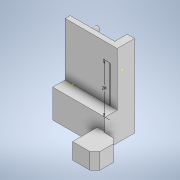
# Autodesk Inventor part: base_fin_carrera
Saved by Autodesk Inventor 2021 (Build 250183000, 183)
## iProperties
Created: 2021-05-13
Part Number: base_fin_carrera
Material: Genérico
Document SubType Name: Modeling
Designer: orgyn
Density: 1 g/cm^3
Appearance: Valor por defecto
Author: orgyn
Autodesk Inventor part; units mm, degrees
ref_plane "YZ Plane" through (0, 0, 0) normal (1, 0, 0) x (0, 1, 0)
ref_plane "XZ Plane" through (0, 0, 0) normal (0, 1, 0) x (-1, 0, 0)
sketch "Boceto1" plane through (0, 0, 0) normal (0, 1, 0) x (-1, 0, 0)
  line L0 (0, 0) -> (-4, 0)
  line L1 (-4, 0) -> (-4, -9.5)
  line L2 (-4, -9.5) -> (0, -9.5)
  line L3 (0, -9.5) -> (0, 0)
  dimension "d0" = 4
  dimension "d1" = 9.5
  constraints: 8 end point, 2 parallel, 1 horizontal, 1 perpendicular
  measures "d0" distance of L2.end L1.end
  measures "d1" distance of L1.end L0.end
extrude "Extrusión1" add sketch "Boceto1" along normal blind 4
sketch "Boceto2" plane through (0, 0, -9.5) normal (-1, 0, 0) x (0, 0, 1)
  line L0 (9.5, 4) -> (0, 4) projected
  line L1 (9.5, 4) -> (-4.5, 4)
  line L2 (-4.5, 4) -> (-7.5, 4)
  line L3 (-5, 0) -> (-5, -16)
  line L4 (0, 0) -> (0, 4) projected
  line L5 (9.5, 0) -> (0, 0) projected
  line L6 (0, 0) -> (9.5, 0)
  line L7 (9.5, 0) -> (9.5, 4)
  line L8 (-5, -16) -> (-12.5, -16)
  line L9 (-12.5, -16) -> (-12.5, 4)
  line L10 (-12.5, 4) -> (-7.5, 4)
  line L11 (-5, 0) -> (9.5, 0)
  line L12 (-5, 4) -> (9.5, 4)
  line L13 (9.5, 0) -> (9.5, 4) projected
  line L14 (9.5, 0) -> (9.5, 4)
  dimension "d4" = 14
  dimension "d5" = 3
  dimension "d6" = 20
  dimension "d25" = 7.5
  constraints: 22 end point, 4 collinear, 3 horizontal, 3 perpendicular
  measures "d4" distance of L0.start L1.end
  measures "d5" distance of L2.end L1.end
  measures "d6" distance of L12.start L3.end
  measures "d25" distance of L8.start L8.end
extrude "Extrusión2" add sketch "Boceto2" along normal blind 2 contours L7 L5 L4 L0
sketch "Boceto3" plane through (-2, 0, -9.5) normal (-1, 0, 0) x (0, 0, 1)
  line L0 (9.5, 4) -> (0, 4) projected
  line L1 (-7.5, 4) -> (-2.5, 4)
  line L2 (-2.5, 4) -> (-2.5, 1.5)
  line L3 (-2.5, 1.5) -> (-7.5, 1.5)
  line L4 (-7.5, 4) -> (-7.5, -16) projected
  line L5 (-7.5, 1.5) -> (-7.5, -4.5)
  line L6 (-7.5, -4.5) -> (-7.5, -10.5)
  line L7 (-7.5, -10.5) -> (-7.5, -13)
  line L8 (-7.5, -13) -> (-2.5, -13)
  line L9 (-2.5, -13) -> (-2.5, -10.5)
  line L10 (-2.5, -10.5) -> (-7.5, -10.5)
  line L11 (-7.5, -4.5) -> (-7.5, -5.75)
  line L12 (-7.5, -5.75) -> (-2.5, -5.75)
  line L13 (-2.5, -5.75) -> (-2.5, -3.25)
  line L14 (-2.5, -3.25) -> (-7.5, -3.25)
  point P0 (9.5, 0)
  dimension "d9" = 5
  dimension "d10" = 2.5
  dimension "d11" = 6
  dimension "d12" = 6
  dimension "d13" = 2.5
  dimension "d14" = 5
  dimension "d15" = 2.5
  dimension "d16" = 1.25
  dimension "d17" = 5
  dimension "d18" = 2.5
  constraints: 26 end point, 9 point on line, 4 perpendicular, 1 parallel
  measures "d9" distance of L1.start L1.end
  measures "d10" distance of L1.end L2.end
  measures "d11" distance of L3.end L5.end
  measures "d12" distance of L5.end L6.end
  measures "d13" distance of L6.end L7.end
  measures "d14" distance of L7.end L8.end
  measures "d15" distance of L8.end L9.end
  measures "d16" distance of L5.end L11.end
  measures "d17" distance of L11.end L12.end
  measures "d18" distance of L12.end L13.end
extrude "Extrusión3" cut sketch "Boceto3" against normal blind 1
chamfer "Chaflán1" distance 2 angle 45 2 edges at (4, 2, -9.5) (4, 2, 0)
sketch "Boceto4" plane through (-2, 0, -9.5) normal (-1, 0, 0) x (0, 0, 1)
  line L0 (0, 0) -> (9.5, 0) projected
  line L1 (9.5, 0) -> (0, 0)
  line L2 (0, 0) -> (-5, 0)
  line L3 (-5, 0) -> (-5, -20)
  line L4 (-5, -20) -> (-12.5, -20)
  line L5 (-12.5, -20) -> (-12.5, 4)
  line L6 (9.5, 4) -> (0, 4) projected
  line L7 (-12.5, 4) -> (9.5, 4)
  line L8 (9.5, 0) -> (9.5, 4) projected
  line L9 (9.5, 4) -> (9.5, 0)
  line L10 (-12.5, 4) -> (-7.5, 4)
  line L11 (-7.5, 4) -> (-7.5, 1.5)
  line L12 (-7.5, 1.5) -> (-12.5, 1.5)
  line L13 (-12.5, 1.2493) -> (-12.5, -4.7507)
  line L14 (-12.5, -4.7507) -> (-12.5, -10.7507)
  line L15 (-12.5, -10.7507) -> (-7.5, -10.7507)
  line L16 (-7.5, -10.7507) -> (-7.5, -13.2507)
  line L17 (-7.5, -13.2507) -> (-12.5, -13.2507)
  line L18 (-12.5, -4.7507) -> (-12.5, -6.0007)
  line L19 (-12.5, -6.0007) -> (-7.5, -6.0007)
  line L20 (-7.5, -6.0007) -> (-7.5, -3.5007)
  line L21 (-7.5, -3.5007) -> (-12.5, -3.5007)
  dimension "d26" = 5
  dimension "d27" = 20
  dimension "d28" = 7.5
  dimension "d29" = 5
  dimension "d30" = 2.5
  dimension "d31" = 6
  dimension "d32" = 6
  dimension "d33" = 5
  dimension "d34" = 2.5
  dimension "d35" = 1.25
  dimension "d36" = 2.5
  constraints: 38 end point, 13 point on line, 8 perpendicular, 3 collinear
  measures "d26" distance of L0.start L2.end
  measures "d27" distance of L2.end L3.end
  measures "d28" distance of L3.end L4.end
  measures "d29" distance of L5.end L10.end
  measures "d30" distance of L10.end L11.end
  measures "d31" distance of L13.start L13.end
  measures "d32" distance of L13.end L14.end
  measures "d33" distance of L14.end L15.end
  measures "d34" distance of L15.end L16.end
  measures "d35" distance of L13.end L18.end
  measures "d36" distance of L19.end L20.end
extrude "Extrusión4" add sketch "Boceto4" along normal blind 3 contours L2 L3 L4 L5 L17 L16 L15 L19 L20 L21 L12 L11 L7 L6 L8 L0
sketch "Boceto5" plane through (0, 4, 0) normal (0, 1, 0) x (1, 0, 0)
  line L0 (-2, 17) -> (-5, 17) projected
  line L1 (-5, 17) -> (-2, 17)
  line L2 (-2, 14.5) -> (-2, 9.5) projected
  line L3 (-2, 17) -> (-2, 9.5)
  line L4 (2, 9.5) -> (-2, 9.5) projected
  line L5 (-2, 9.5) -> (2, 9.5)
  line L6 (4, 7.5) -> (2, 9.5) projected
  line L7 (2, 9.5) -> (4, 7.5)
  line L8 (4, 2) -> (4, 7.5) projected
  line L9 (4, 7.5) -> (4, 2)
  line L10 (2, 0) -> (4, 2) projected
  line L11 (4, 2) -> (2, 0)
  line L12 (2, 0) -> (-5, 0) projected
  line L13 (2, 0) -> (-5, 0)
  line L14 (-5, 0) -> (-5, 17) projected
  line L15 (-5, 0) -> (-5, 17)
  point P0 (0, 0)
  constraints: 16 end point, 4 collinear, 3 perpendicular, 1 parallel
extrude "Extrusión5" add sketch "Boceto5" along normal blind 2.5
sketch "Boceto7" plane through (-5, 0, -9.5) normal (-1, 0, 0) x (0, 0, 1)
  line L0 (-7.5, 1.5) -> (-7.5, 6.5) projected
  line L1 (-7.5, 1.5) -> (-7.5, -20)
  line L2 (-12.5, -20) -> (-5, -20) projected
  line L3 (-7.5, -20) -> (-5.5, -20)
  line L4 (-5.5, -20) -> (-5.5, 6.5)
  line L5 (0, 6.5) -> (-7.5, 6.5) projected
  line L6 (-7.5, 6.5) -> (-7.5, 1.5)
  point P0 (9.5, 0)
  dimension "d41" = 2
  constraints: 8 end point, 3 point on line, 1 parallel, 1 vertical
  measures "d41" distance of L1.end L3.end
extrude "Extrusión6" add sketch "Boceto7" along normal blind 8
sketch "Boceto8" plane through (-2, -13.2507, -17) normal (0, 0, -1) x (-1, 0, 0)
  line L0 (0, 14.7507) -> (0, 19.7507) projected
  line L1 (0, 14.7507) -> (2, 14.7507)
  line L2 (2, 14.7507) -> (6, 14.7507)
  line L3 (6, 14.7507) -> (6, 19.7507)
  line L4 (3, 19.7507) -> (11, 19.7507) projected
  circle A0 centre (6, 14.7507) radius 1
  line L5 (6, 13.7507) -> (6, 7.7507)
  line L6 (6, 7.7507) -> (6, 6.1507)
  circle A1 centre (6, 6.1507) radius 1
  line L7 (6, 6.1507) -> (5.7406, 6.1507)
  point P0 (-2, 13.2507)
  dimension "d46" = 2
  dimension "d44" = 2
  dimension "d45" = 4
  dimension "d47" = 6
  constraints: 12 end point, 2 coincident, 2 horizontal, 2 point on line, 2 vertical, 1 centre point, 1 perpendicular, 1 vertical alignment, 2 other
  measures "d44" distance of L0.start L1.end
  measures "d45" distance of L1.end L2.end
  measures "d47" distance of L5.start L5.end
extrude "Extrusión7" add sketch "Boceto8" along normal blind 6
sketch "Boceto9" plane through (-2, -20, -14.5) normal (0, 0, 1) x (1, 0, 0)
  line L0 (0, 0) -> (0, 20) projected
  line L1 (0, 20) -> (-3, 20) projected
  line L2 (0, 20) -> (-3, 20)
  line L3 (-3, 0) -> (-11, 0) projected
  line L4 (-3, 20) -> (-3, 0)
  line L5 (0, 0) -> (-3, 0) projected
  line L6 (-3, 0) -> (0, 0)
  line L7 (0, 0) -> (0, 20)
  point P0 (2, 20)
  constraints: 8 end point, 3 perpendicular, 1 collinear
extrude "Extrusión8" cut sketch "Boceto9" against normal blind 0.5
sketch "Boceto10" plane through (-2, -3.5007, -22) normal (0, 0, -1) x (-1, 0, 0)
  line L0 (0, 5.0007) -> (3, 5.0007) projected
  line L1 (0, 5.0007) -> (0, 0) projected
  line L2 (3, 5.0007) -> (0, 5.0007)
  line L3 (0, 5.0007) -> (0, 0)
  line L4 (0, 0) -> (3, 0)
  line L5 (3, 0) -> (3, 5.0007)
  line L6 (0, -2.5) -> (3, -2.5) projected
  line L7 (0, -7.25) -> (3, -7.25) projected
  line L8 (3, -2.5) -> (0, -2.5)
  line L9 (0, -2.5) -> (0, -7.25)
  line L10 (0, -7.25) -> (3, -7.25)
  line L11 (3, -7.25) -> (3, -2.5)
  line L12 (3, -16.4993) -> (3, -9.75) projected
  line L13 (0, 3.5007) -> (0, -16.4993) projected
  line L14 (3, -9.75) -> (0, -9.75)
  line L15 (0, -9.75) -> (0, -16.4993)
  line L16 (0, -16.4993) -> (3, -16.4993)
  line L17 (3, -16.4993) -> (3, -9.75)
  point P0 (-2, 3.5007)
  constraints: 24 end point, 6 parallel, 3 horizontal, 3 perpendicular
extrude "Extrusión9" cut sketch "Boceto10" against normal blind 5
sketch "Boceto11" plane through (-5, 0, -15) normal (0, 0, 1) x (1, 0, 0)
  line L0 (0, 0) -> (0, -20)
  point P0 (5, 0)
  dimension "d58" = 20
  constraints: 2 end point, 1 vertical
  measures "d58" distance of L0.start L0.end
ref_plane "Plano de trabajo1" through (0, -10, 0) normal (0, -1, 0) x (1, 0, 0)
mirror "Simetría1" about plane through (0, -10, 0) normal (0, -1, 0) of "Extrusión5"
sketch "Boceto12" plane through (-5, -24, 0) normal (0, 1, 0) x (1, 0, 0)
  line L0 (0, 0) -> (7, 0) projected
  line L1 (0, 17) -> (0, 0) projected
  line L2 (0, 0) -> (0, 17)
  line L3 (3, 9.5) -> (3, 17) projected
  line L4 (0, 17) -> (3, 17)
  line L5 (3, 17) -> (3, 9.5)
  line L6 (7, 9.5) -> (3, 9.5) projected
  line L7 (3, 9.5) -> (7, 9.5)
  line L8 (9, 7.5) -> (7, 9.5) projected
  line L9 (7, 9.5) -> (9, 7.5)
  line L10 (9, 2) -> (9, 7.5) projected
  line L11 (9, 7.5) -> (9, 2)
  line L12 (9, 2) -> (7, 0)
  line L13 (7, 0) -> (0, 0)
  point P0 (5, 0)
  constraints: 16 end point, 4 collinear, 2 perpendicular, 1 parallel, 1 vertical
extrude "Extrusión10" add sketch "Boceto12" along normal blind 4
sketch "Boceto13" plane through (0, 6.5, 0) normal (0, 1, 0) x (1, 0, 0)
  line L0 (-5, 15) -> (-2, 15) projected
  line L1 (-5, 15) -> (10.3969, 15)
  line L2 (10.3969, 15) -> (10.0462, -8.8687)
  line L3 (10.0462, -8.8687) -> (-11.5494, -8.8687)
  line L4 (-11.5494, -8.8687) -> (-11.5494, 15)
  line L5 (-5, 15) -> (-13, 15) projected
  line L6 (-5, 15) -> (-11.5494, 15)
  point P0 (0, 0)
  constraints: 10 end point, 2 perpendicular, 1 horizontal, 1 parallel, 1 point on line
extrude "Extrusión11" cut sketch "Boceto13" against normal blind 9
sketch "Boceto14" plane through (-13, -20, -17) normal (0, -1, 0) x (1, 0, 0)
  line L0 (11, 0) -> (0, 0) projected
  line L1 (8, 2) -> (0, 2) projected
  line L2 (0, 0) -> (8, 0)
  line L3 (8, 0) -> (8, 2)
  line L4 (8, 2) -> (0, 2)
  line L5 (0, 2) -> (0, 0)
  point P0 (13, 17)
  constraints: 8 end point, 2 parallel, 1 horizontal, 1 perpendicular
extrude "Extrusión12" add sketch "Boceto14" along normal blind 6.5
sketch "Boceto15" plane through (-2, 6.5, -17) normal (0, 0, -1) x (-1, 0, 0)
  line L0 (0, 0) -> (11, 0) projected
  line L1 (5.9919, 0) -> (15.9919, 0)
  line L2 (15.9919, 0) -> (15.9919, -33)
  circle A0 centre (6, -5) radius 1 projected
  line L3 (6, -5) -> (25.1824, -5)
  circle A1 centre (6, -13.6) radius 1 projected
  line L4 (6, -13.6) -> (25.934, -13.6)
  circle A2 centre (15.9919, -5) radius 1
  circle A3 centre (15.967, -13.6) radius 1
  line L5 (11, 0) -> (21, 0)
  line L6 (21, 0) -> (21, -33)
  line L7 (11, 0) -> (11, -33) projected
  line L8 (21, -33) -> (11, -33)
  line L9 (11, -33) -> (11, 0)
  point P0 (-2, -6.5)
  dimension "d66" = 10
  dimension "d67" = 2
  dimension "d68" = 2
  dimension "d69" = 10
  constraints: 16 end point, 4 perpendicular, 4 point on line, 2 centre point, 2 horizontal, 1 collinear, 1 midpoint
  measures "d66" distance of L1.start L1.end
  measures "d67" diameter of A2
  measures "d68" diameter of A3
  measures "d69" distance of L0.end L5.end
extrude "Extrusión13" add sketch "Boceto15" against normal blind 2 contours L1 L2 A2 L3 L7 | L5 L6 L3 A2 L2 | L3 A2 L2 A3 L4 L7 | A2 L3 L2 | L2 L3 A2 | L3 L2 A2 | L4 A3 L2 L8 L7 | L3 A2 L2 | L3 L6 L4 A3 L2 A2 | A3 L2 L4 | L4 L2 A3 | L6 L8 L2 A3 L4 | A3 L4 L2 | L4 A3 L2
sketch "Boceto16" plane through (-2, -26.5, -17) normal (0, 0, -1) x (-1, 0, 0)
  circle A0 centre (6, 28) radius 1 projected
  line L0 (6, 28) -> (16, 28)
  circle A1 centre (6, 19.4) radius 1 projected
  line L1 (6, 19.4) -> (16, 19.4)
  circle A2 centre (16, 28) radius 1
  circle A3 centre (16, 19.4) radius 1
  point P0 (-2, 26.5)
  dimension "d72" = 10
  dimension "d73" = 10
  dimension "d74" = 2
  dimension "d75" = 2
  constraints: 4 end point, 2 centre point, 2 coincident, 2 horizontal
  measures "d72" distance of L0.start L0.end
  measures "d73" distance of L1.start L1.end
  measures "d74" diameter of A2
  measures "d75" diameter of A3
extrude "Extrusión14" add sketch "Boceto16" along normal blind 6 contours A2 | A3
sketch "Boceto17" plane through (-8, -7.1, -23) normal (0, 0, -1) x (-1, 0, 0)
  line L0 (4.3511, -2.3199) -> (4.3511, 11.9603)
  line L1 (4.3511, 11.9603) -> (-3.8663, 11.9603)
  line L2 (-3.8663, 11.9603) -> (-3.8663, -2.9713)
  line L3 (-3.8663, -2.9713) -> (4.3511, -2.3199)
  point P0 (-8, 7.1)
  constraints: 8 end point, 2 perpendicular, 1 vertical
extrude "Extrusión15" cut sketch "Boceto17" against normal blind 6
sketch "Boceto18" plane through (-2, -26.5, -17) normal (0, 0, -1) x (-1, 0, 0)
  line L0 (3, 6.5) -> (3, 0) projected
  line L1 (0, 0) -> (3, 0)
  line L2 (3, 0) -> (3, 33)
  line L3 (0, 33) -> (21, 33) projected
  line L4 (0, 33) -> (21, 33) projected
  line L5 (3, 33) -> (0, 33)
  line L6 (0, 33) -> (0, 0)
  line L7 (3, 0) -> (-4, 0) projected
  line L8 (-4, 0) -> (0, 0) projected
  line L9 (3, 0) -> (0, 0)
  line L10 (1.5, 33) -> (1.5, 0)
  line L11 (1.5, 33) -> (1.5, 23)
  circle A0 centre (1.5, 23) radius 1
  line L12 (1.5, 0) -> (1.5, 10)
  circle A1 centre (1.5, 10) radius 1
  point P0 (-2, 26.5)
  dimension "d82" = 10
  dimension "d83" = 2
  dimension "d84" = 10
  dimension "d85" = 2
  constraints: 16 end point, 3 point on line, 2 centre point, 2 horizontal, 2 midpoint, 2 perpendicular, 1 coincident, 1 collinear
  measures "d82" distance of L10.start L11.end
  measures "d83" diameter of A0
  measures "d84" distance of L10.end L12.end
  measures "d85" diameter of A1
extrude "Extrusión16" add sketch "Boceto18" along normal blind 5 contours L0 L1 L10 A1 A0 L3 L2 | L1 L6 L3 L10 A0 A1
sketch "Boceto19" plane through (-5, -20, -15) normal (0, 0, 1) x (1, 0, 0)
  line L0 (3, 0) -> (-18, 0)
  line L1 (-18, 26.5) -> (-18, -6.5) projected
  line L2 (-18, 0) -> (-18, 5)
  line L3 (-18, 5) -> (2.826, 5)
  line L4 (2.826, 5) -> (3, 5)
  line L5 (3, 26.5) -> (3, 0) projected
  line L6 (3, 5) -> (3, 0)
  point P0 (5, 20)
  dimension "d86" = 5
  constraints: 10 end point, 2 horizontal, 2 perpendicular, 2 point on line
  measures "d86" distance of L0.end L2.end
extrude "Extrusión17" add sketch "Boceto19" along normal blind 5
sketch "Boceto20" plane through (-23, -20, -15) normal (0, -1, 0) x (1, 0, 0)
  line L0 (0, 0) -> (0, 5) projected
  line L1 (0, 5) -> (18, 5) projected
  line L2 (0, 0) -> (18, 0)
  line L3 (18, 0) -> (18, 5)
  line L4 (18, 5) -> (0, 5)
  line L5 (0, 5) -> (0, 0)
  point P0 (23, 15)
  constraints: 8 end point, 2 parallel, 1 horizontal, 1 perpendicular
extrude "Extrusión18" add sketch "Boceto20" along normal blind 6.5
sketch "Boceto21" plane through (-5, -26.5, -17) normal (-1, 0, 0) x (0, 0, 1)
  point P0 (17, 26.5)
